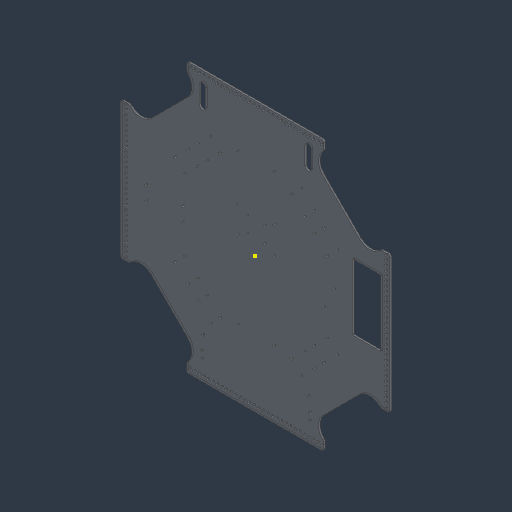
# Autodesk Inventor part: BellyPanTop
Saved by Autodesk Inventor 2024.3 (Build 283343000, 343)
## iProperties
Created: 2025-01-13
Part Number: BellyPanTop
Material: Lexan, Clear
Document SubType Name: Sheet Metal
Designer: Marcus Tannini
Density: 1.2 g/cm^3
Appearance: Lexan (Clear)
Mfg Approved By: John.Thibert
Sheet Metal Rule: Default
Mass: 2396.13 g
Surface Area: 8683.97 cm^2
Volume: 1996.77 cm^3
ILogicPurgeVersion: 0.0.0.0
OnSaveVersion: 3.5.0.0
OnSaveAssembly: COREAutomationManager
ModelCat: Uncategorized
MaterialName: Lexan, Clear
CN_MASS: 2.4
Author: Marcus Tannini
Autodesk Inventor part; units mm, degrees
ref_plane "YZ Plane" through (0, 0, 0) normal (1, 0, 0) x (0, 1, 0)
ref_plane "XZ Plane" through (0, 0, 0) normal (0, 1, 0) x (-1, 0, 0)
ref_plane "XY Plane" through (0, 0, 0) normal (0, 0, 1) x (1, 0, 0)
sketch "Sketch5" plane through (0, 0, 0) normal (0, 0, 1) x (1, 0, 0)
  line L0 (-374.65, 374.65) -> (374.65, 374.65)
  line L1 (374.65, 374.65) -> (374.65, -374.65)
  line L2 (374.65, -374.65) -> (-374.65, -374.65)
  line L3 (-374.65, -374.65) -> (-374.65, 374.65)
  line L4 (-374.65, 374.65) -> (374.65, -374.65) construction
  line L5 (374.65, 374.65) -> (-374.65, -374.65) construction
  line L6 (374.65, 190.5) -> (349.25, 190.5)
  arc A0 (289.7334, 187.4984) -> (349.25, 190.5) centre (318.135, 215.9) ccw
  line L7 (289.7334, 187.4984) -> (187.4984, 289.7334)
  line L8 (190.5, 374.65) -> (190.5, 349.25)
  arc A1 (190.5, 349.25) -> (187.4984, 289.7334) centre (215.9, 318.135) ccw
  point P0 (0, 0)
  point P1 (238.6159, 238.6159)
  dimension "d22" = 749.3
  dimension "d23" = 749.3
  dimension "d24" = 184.15
  dimension "d27" = 25.4
  dimension "d29" = 40.166
  dimension "d31" = 158.75
  constraints: 18 end point, 4 point on circle, 3 midpoint, 3 perpendicular, 3 symmetric about line, 2 centre point, 2 parallel, 2 point on line, 1 horizontal, 1 tangent, 1 other
  measures "d22" distance of L1.end L2.end
  measures "d23" distance of L0.end L1.end
  measures "d24" distance between parallel lines of L0 L6
  measures "d27" distance of L6.start L6.end
  measures "d29" radius of A0
  measures "d31" distance from line of L0 A0.centre
extrude "Plate1" add sketch "Sketch5" along normal mid plane 4.7625
extrude "Extrusion3" cut sketch "Sketch5" along normal through all both and the other way through all contours L0 L1 L6 A0 L7 A1 L8
fillet "Corner Round1" radius 6.35 2 edges at (349.25, 190.5, 0) (190.5, 349.25, 0)
pattern_circular "Circular Pattern1" count 4 over 360 about axis through (0, 0, -10) along (0, 0, 1) of "Extrusion3", "Corner Round1"
fillet "Corner Round2" radius 6 8 edges at (374.65, 190.5, 0) (190.5, 374.65, 0) (-190.5, 374.65, 0) (-374.65, 190.5, 0) (-374.65, -190.5, 0) (-190.5, -374.65, 0) (190.5, -374.65, 0) (374.65, -190.5, 0)
sketch "Sketch6" plane through (0, 0, -2.3813) normal (0, 0, -1) x (-1, 0, 0)
  line L0 (-352.1302, 190.5) -> (-368.65, 190.5) construction
  line L1 (-374.65, -184.5) -> (-374.65, 184.5) construction
  point P0 (0, 0)
  point P1 (-361.95, 184.15)
  dimension "d40" = 6.35
  dimension "d41" = 12.7
  measures "d40" distance from line of L0 point (-361.95, 184.15)
  measures "d41" distance from line of point (-361.95, 184.15) L1
hole "Hole1" at (361.95, 184.15, -2.3813) direction (0, 0, 1) diameter 5.1054 end through all clearance for "Flat Head Machine Screw (82)" size "#10" standard "Ansi Unified Screw Threads"
sketch "Sketch8" plane through (0, 0, 2.3813) normal (0, 0, 1) x (1, 0, 0)
  line L0 (162.2837, -189.2245) -> (126.3627, -225.1455) construction
  line L1 (126.3627, -225.1455) -> (99.4219, -198.2047) construction
  line L2 (99.4219, -198.2047) -> (135.3429, -162.2837) construction
  line L3 (135.3429, -162.2837) -> (162.2837, -189.2245) construction
  line L4 (162.2837, -189.2245) -> (99.4219, -198.2047) construction
  line L5 (126.3627, -225.1455) -> (135.3429, -162.2837) construction
  line L6 (187.4984, -289.7334) -> (289.7334, -187.4984) construction
  line L7 (238.6159, -238.6159) -> (0, 0) construction
  line L8 (189.2245, -162.2837) -> (225.1455, -126.3627) construction
  line L9 (225.1455, -126.3627) -> (198.2047, -99.4219) construction
  line L10 (198.2047, -99.4219) -> (162.2837, -135.3429) construction
  line L11 (162.2837, -135.3429) -> (189.2245, -162.2837) construction
  line L12 (189.2245, -162.2837) -> (198.2047, -99.4219) construction
  line L13 (225.1455, -126.3627) -> (162.2837, -135.3429) construction
  point P0 (130.8528, -193.7146)
  point P1 (193.7146, -130.8528)
  point P2 (130.8528, -193.7146)
  point P3 (130.8528, -193.7146)
  dimension "d65" = 38.1
  dimension "d66" = 50.8
  dimension "d79" = 88.9
  dimension "d80" = 38.1
  constraints: 26 end point, 8 coincident, 7 midpoint, 4 parallel, 4 perpendicular, 2 equal length, 1 symmetric about line
  measures "d65" distance of L2.end L0.start
  measures "d66" distance of L0.start L0.end
  measures "d79" distance between parallel lines of L6 L0
  measures "d80" distance between parallel lines of L11 L3
hole "Hole2" at (135.3429, -162.2837, 2.3813) at (162.2837, -189.2245, 2.3813) at (126.3627, -225.1455, 2.3813) at (99.4219, -198.2047, 2.3813) at (162.2837, -135.3429, 2.3813) at (189.2245, -162.2837, 2.3813) at (225.1455, -126.3627, 2.3813) at (198.2047, -99.4219, 2.3813) direction (0, 0, -1) diameter 3.9624 end through all start extended yes thread size "10-32 UNF" class "2B" standard "ANSI Unified Screw Threads"
pattern_linear "Rectangular Pattern1" count 30 spacing 12.7 along (0, -1, 0) of "Hole1"
pattern_circular "Circular Pattern2" count 4 over 360 about axis through (0, 0, -10) along (0, 0, 1) of "Hole1", "Rectangular Pattern1", "Hole2"
sketch "Sketch9" plane through (0, 0, 2.3813) normal (0, 0, 1) x (1, 0, 0)
  line L0 (217.17, 28.575) -> (217.17, -28.575) construction
  line L1 (217.17, -28.575) -> (189.23, -28.575) construction
  line L2 (189.23, -28.575) -> (189.23, 28.575) construction
  line L3 (189.23, 28.575) -> (217.17, 28.575) construction
  line L4 (217.17, 28.575) -> (189.23, -28.575) construction
  line L5 (217.17, -28.575) -> (189.23, 28.575) construction
  line L6 (0, 524.51) -> (0, -524.51) construction
  line L7 (-524.51, 0) -> (524.51, 0) construction
  point P0 (0, 0)
  point P1 (203.2, 0)
  point P2 (203.2, 0)
  dimension "d81" = 57.15
  dimension "d82" = 27.94
  dimension "d166" = 203.2
  constraints: 12 end point, 2 coincident, 2 midpoint, 2 parallel, 1 perpendicular, 1 point on line
  measures "d81" distance of L1.end L2.end
  measures "d82" distance of L2.end L0.start
  measures "d166" distance from line of L6 point (203.2, 0)
hole "Main Breaker" at (217.17, 28.575, 2.3813) at (189.23, -28.575, 2.3813) direction (0, 0, -1) diameter 3.9624 end through all start extended yes thread size "10-32 UNF" class "2B" standard "ANSI Unified Screw Threads"
sketch "Sketch10" plane through (0, 0, 2.3813) normal (0, 0, 1) x (1, 0, 0)
  line L0 (0, 524.51) -> (0, -524.51) construction
  line L1 (50.8, -190.5) -> (-50.8, -190.5) construction
  line L2 (-50.8, -190.5) -> (-50.8, 25.4) construction
  line L3 (-50.8, 25.4) -> (50.8, 25.4) construction
  line L4 (50.8, 25.4) -> (50.8, -190.5) construction
  line L5 (50.8, -190.5) -> (-50.8, 25.4) construction
  line L6 (-50.8, -190.5) -> (50.8, 25.4) construction
  point P0 (0, 0)
  point P1 (0, -82.55)
  dimension "d91" = 101.6
  dimension "d92" = 25.4
  dimension "d93" = 215.9
  constraints: 12 end point, 4 coincident, 2 midpoint, 2 parallel, 1 horizontal, 1 perpendicular, 1 point on line
  measures "d91" distance of L2.end L3.end
  measures "d92" distance from line of point (0, 0) L3
  measures "d93" distance of L1.end L2.end
hole "PDP" at (-50.8, 25.4, 2.3813) at (50.8, 25.4, 2.3813) at (50.8, -190.5, 2.3813) at (-50.8, -190.5, 2.3813) direction (0, 0, -1) diameter 3.9624 end through all start extended yes thread size "10-32 UNF" class "2B" standard "ANSI Unified Screw Threads"
sketch "Sketch11" plane through (0, 0, 2.3813) normal (0, 0, 1) x (1, 0, 0)
  line L0 (23.876, 41.9735) -> (-23.876, 41.9735) construction
  line L1 (-23.876, 41.9735) -> (-23.876, 85.0265) construction
  line L2 (-23.876, 85.0265) -> (23.876, 85.0265) construction
  line L3 (23.876, 85.0265) -> (23.876, 41.9735) construction
  line L4 (23.876, 41.9735) -> (-23.876, 85.0265) construction
  line L5 (-23.876, 41.9735) -> (23.876, 85.0265) construction
  line L6 (0, 524.51) -> (0, -524.51) construction
  line L7 (-524.51, 0) -> (524.51, 0) construction
  point P0 (0, 0)
  point P1 (0, 63.5)
  dimension "d101" = 43.053
  dimension "d102" = 47.752
  dimension "d103" = 63.5
  constraints: 12 end point, 4 coincident, 2 midpoint, 2 parallel, 1 horizontal, 1 perpendicular, 1 point on line
  measures "d101" distance of L0.end L1.end
  measures "d102" distance of L1.end L2.end
  measures "d103" distance from line of L7 point (0, 63.5)
hole "VRM" at (-23.876, 85.0265, 2.3813) at (-23.876, 41.9735, 2.3813) at (23.876, 85.0265, 2.3813) at (23.876, 41.9735, 2.3813) direction (0, 0, -1) diameter 3.302 end through all start extended yes thread size "8-32 UNC" class "2B" standard "ANSI Unified Screw Threads"
sketch "Sketch12" plane through (0, 0, -2.3813) normal (0, 0, -1) x (-1, 0, 0)
  line L0 (-50.8, 228.6) -> (50.8, 228.6) construction
  line L1 (50.8, 228.6) -> (50.8, 101.6) construction
  line L2 (50.8, 101.6) -> (-50.8, 101.6) construction
  line L3 (-50.8, 101.6) -> (-50.8, 228.6) construction
  line L4 (-50.8, 228.6) -> (50.8, 101.6) construction
  line L5 (50.8, 228.6) -> (-50.8, 101.6) construction
  line L6 (0, -524.51) -> (0, 524.51) construction
  point P0 (0, 0)
  point P1 (0, 165.1)
  dimension "d111" = 165.1
  dimension "d112" = 101.6
  dimension "d113" = 127
  constraints: 12 end point, 4 coincident, 2 midpoint, 2 parallel, 1 horizontal, 1 perpendicular, 1 point on line
  measures "d111" distance of point (0, 0) point (0, 165.1)
  measures "d112" distance of L1.end L2.end
  measures "d113" distance of L0.end L1.end
hole "RoboRIO" at (-50.8, 101.6, -2.3813) at (50.8, 101.6, -2.3813) at (50.8, 228.6, -2.3813) at (-50.8, 228.6, -2.3813) direction (0, 0, 1) diameter 2.9464 end through all start extended yes clearance for "Socket Head Cap Screw" size "#4" standard "Ansi Unified Screw Threads"
sketch "Sketch13" plane through (0, 0, 2.3813) normal (0, 0, 1) x (1, 0, 0)
  line L0 (-203.2, -19.05) -> (-304.8, -19.05) construction
  line L1 (-304.8, -19.05) -> (-304.8, 19.05) construction
  line L2 (-304.8, 19.05) -> (-203.2, 19.05) construction
  line L3 (-203.2, 19.05) -> (-203.2, -19.05) construction
  line L4 (-203.2, -19.05) -> (-304.8, 19.05) construction
  line L5 (-304.8, -19.05) -> (-203.2, 19.05) construction
  line L6 (-524.51, 0) -> (524.51, 0) construction
  point P0 (0, 0)
  point P1 (-254, 0)
  dimension "d121" = 101.6
  dimension "d122" = 38.1
  dimension "d149" = 254
  constraints: 12 end point, 4 coincident, 2 midpoint, 2 parallel, 1 horizontal, 1 perpendicular, 1 point on line
  measures "d121" distance of L1.end L2.end
  measures "d122" distance of L0.end L1.end
  measures "d149" distance of point (0, 0) point (-254, 0)
hole "Pneumatics Hub" at (-304.8, 19.05, 2.3813) at (-203.2, 19.05, 2.3813) at (-203.2, -19.05, 2.3813) at (-304.8, -19.05, 2.3813) direction (0, 0, -1) diameter 3.9624 end through all start extended yes thread size "10-32 UNF" class "2B" standard "ANSI Unified Screw Threads"
sketch "Sketch7" plane through (0, 0, -2.3813) normal (0, 0, -1) x (-1, 0, 0)
  line L0 (0, -524.51) -> (0, 524.51) construction
  line L1 (-524.51, 0) -> (524.51, 0) construction
  line L2 (-349.25, -53.975) -> (-270.51, -53.975)
  line L3 (-270.51, -53.975) -> (-270.51, 130.175)
  line L4 (-270.51, 130.175) -> (-349.25, 130.175)
  line L5 (-349.25, 130.175) -> (-349.25, -53.975)
  line L6 (-349.25, -53.975) -> (-270.51, 130.175) construction
  line L7 (-270.51, -53.975) -> (-349.25, 130.175) construction
  point P0 (0, 0)
  dimension "d133" = 78.74
  dimension "d134" = 184.15
  dimension "d165" = 349.25
  dimension "d168" = 53.975
  constraints: 12 end point, 2 parallel, 1 horizontal, 1 perpendicular
  measures "d133" distance of L3.end L4.end
  measures "d134" distance of L2.end L3.end
  measures "d165" distance between parallel lines of L5 L0
  measures "d168" distance between parallel lines of L1 L2
extrude "Cut1" cut sketch "Sketch7" against normal blind 4.7625
sketch "Sketch15" plane through (0, 0, 2.3813) normal (0, 0, 1) x (1, 0, 0)
  line L0 (-147.0025, 279.4) -> (-147.0025, 279.4)
  line L1 (-155.8925, 288.29) -> (-155.8925, 336.55)
  line L2 (-147.0025, 345.44) -> (-147.0025, 345.44)
  line L3 (-138.1125, 336.55) -> (-138.1125, 288.29)
  line L4 (-138.1125, 279.4) -> (-155.8925, 345.44) construction
  line L5 (-155.8925, 279.4) -> (-138.1125, 345.44) construction
  line L6 (0, 524.51) -> (0, -524.51) construction
  line L7 (147.0025, 279.4) -> (147.0025, 279.4)
  line L8 (155.8925, 288.29) -> (155.8925, 336.55)
  line L9 (147.0025, 345.44) -> (147.0025, 345.44)
  line L10 (138.1125, 336.55) -> (138.1125, 288.29)
  line L11 (138.1125, 279.4) -> (155.8925, 345.44) construction
  line L12 (155.8925, 279.4) -> (138.1125, 345.44) construction
  line L13 (-524.51, 0) -> (524.51, 0) construction
  arc A0 (147.0025, 279.4) -> (155.8925, 288.29) centre (147.0025, 288.29) ccw
  arc A1 (155.8925, 336.55) -> (147.0025, 345.44) centre (147.0025, 336.55) ccw
  arc A2 (147.0025, 345.44) -> (138.1125, 336.55) centre (147.0025, 336.55) ccw
  arc A3 (138.1125, 288.29) -> (147.0025, 279.4) centre (147.0025, 288.29) ccw
  arc A4 (-147.0025, 279.4) -> (-138.1125, 288.29) centre (-147.0025, 288.29) ccw
  arc A5 (-138.1125, 336.55) -> (-147.0025, 345.44) centre (-147.0025, 336.55) ccw
  arc A6 (-147.0025, 345.44) -> (-155.8925, 336.55) centre (-147.0025, 336.55) ccw
  arc A7 (-155.8925, 288.29) -> (-147.0025, 279.4) centre (-147.0025, 288.29) ccw
  point P0 (0, 0)
  point P1 (-147.0025, 312.42)
  point P2 (147.0025, 312.42)
  dimension "d157" = 17.78
  dimension "d158" = 66.04
  dimension "d159" = 276.225
  dimension "d160" = 279.4
  dimension "d163" = 8.89
  constraints: 24 end point, 16 point on circle, 16 point on line, 16 tangent, 8 centre point, 7 equal radius, 5 symmetric about line, 2 midpoint, 2 parallel, 1 horizontal, 1 perpendicular
  measures "d157" distance of L4.end L5.end
  measures "d158" distance of L5.start L4.end
  measures "d159" distance between parallel lines of L10 L3
  measures "d160" distance between parallel lines of L13 L0
  measures "d163" radius of A0
extrude "Cut2" cut sketch "Sketch15" against normal blind 4.7625
fillet "Corner Round3" radius 1.5875 4 edges at (270.51, 130.175, 0) (349.25, 130.175, 0) (349.25, -53.975, 0) (270.51, -53.975, 0)
sketch "Sketch16" plane through (0, 0, -2.3813) normal (0, 0, -1) x (-1, 0, 0)
  line L0 (155.575, -260.35) -> (155.575, -336.55) construction
  line L1 (138.1125, -336.55) -> (138.1125, -260.35) construction
  line L2 (138.1125, -260.35) -> (155.575, -260.35) construction
  line L3 (138.1125, -336.55) -> (155.575, -336.55) construction
  line L4 (184.5, -374.65) -> (-184.5, -374.65) construction
  line L5 (0, 0) -> (0, -25.4) construction
  circle A0 centre (0, -311.15) radius 149.8282 construction
  line L6 (-149.8283, -301.625) -> (-149.8283, -320.675) construction
  line L7 (-155.575, -260.35) -> (-155.575, -336.55) projected
  point P0 (146.8438, -260.35)
  point P1 (0, -374.65)
  point P2 (-149.8283, -311.15)
  point P3 (149.8283, -301.625)
  point P4 (149.8283, -320.675)
  point P5 (-146.8374, -263.525)
  point P6 (146.8501, -263.525)
  dimension "d178" = 299.6565
  dimension "d170" = 25.4
  dimension "d179" = 63.5
  dimension "d187" = 19.05
  dimension "d188" = 8.7376
  dimension "d189" = 38.1
  dimension "d190" = 8.7376
  dimension "d191" = 38.1
  constraints: 12 end point, 5 vertical, 3 midpoint, 2 coincident, 2 horizontal, 2 symmetric about line, 1 horizontal alignment, 1 vertical alignment, 6 other
  measures "d170" distance of L5.start L5.end
  measures "d179" distance from line of L4 point (0, -311.15)
  measures "d187" distance of L6.start L6.end
  measures "d188" distance from line of L7 point (-146.837, -263.525)
  measures "d189" vertical distance of point (-149.828, -301.625) point (-146.837, -263.525)
  measures "d190" distance from line of L1 point (146.85, -263.525)
  measures "d191" vertical distance of point (149.828, -301.625) point (146.85, -263.525)
hole "Hole11" at (149.8283, -301.625, -2.3813) at (149.8283, -320.675, -2.3813) at (-149.8283, -301.625, -2.3813) at (-149.8283, -320.675, -2.3813) at (146.8374, -263.525, -2.3813) at (-146.8501, -263.525, -2.3813) direction (0, 0, 1) diameter 5.1054 end through all clearance for "Flat Head Machine Screw (82)" size "#10" standard "Ansi Unified Screw Threads"
sketch "Sketch17" plane through (0, 0, 2.3813) normal (0, 0, 1) x (1, 0, 0)
  point P0 (0, 0)
equation "\"d47\" = Thickness"
equation "\"d89\" = Thickness"
equation "\"d63\" = Thickness"
equation "\"d161\" = Thickness"
equation "\"d32\" = Thickness"
equation "\"BendRadius\" = Thickness"
equation "\"BendReliefWidth\" = Thickness"
equation "\"BendReliefDepth\" = 0.5 * Thickness"
equation "\"CornerReliefSize\" = 4 * Thickness"
equation "\"MinimumRemnant\" = 2 * Thickness"
equation "\"TransitionRadius\" = BendRadius"
equation "\"JacobiRadiusSize\" = BendRadius"
equation "\"GapSize\" = Thickness"
equation "\"Thickness\" = 4.7625"
body "Solid2"
